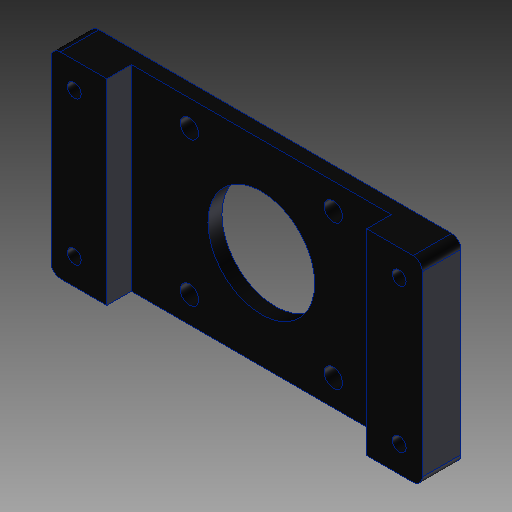
# Autodesk Inventor part: 3217a_Stepper Motor Plate_V1
Saved by Autodesk Inventor 2020 (Build 240168000, 168)
## iProperties
Created: 2019-11-01
Part Number: 3217a_Stepper Motor Plate_V1
Material: Aluminum 6061
Document SubType Name: Modeling
Designer: RFLab
Density: 2.7 g/cm^3
Appearance: Aluminum - Flat
Mass: 37.4548 g
Surface Area: 83.1003 cm^2
Volume: 13.8722 cm^3
Author: RFLab
Autodesk Inventor part; units mm, degrees
ref_plane "YZ Plane" through (0, 0, 0) normal (1, 0, 0) x (0, 1, 0)
ref_plane "XZ Plane" through (0, 0, 0) normal (0, 1, 0) x (-1, 0, 0)
ref_plane "XY Plane" through (0, 0, 0) normal (0, 0, 1) x (1, 0, 0)
sketch "Sketch1" plane through (0, 0, 0) normal (0, 0, 1) x (1, 0, 0)
  line L0 (-40, -21.15) -> (40, -21.15)
  line L1 (40, -21.15) -> (40, 21.15)
  line L2 (40, 21.15) -> (-40, 21.15)
  line L3 (-40, 21.15) -> (-40, -21.15)
  line L4 (-15.5, -15.5) -> (15.5, -15.5) construction
  line L5 (15.5, -15.5) -> (15.5, 15.5) construction
  line L6 (15.5, 15.5) -> (-15.5, 15.5) construction
  line L7 (-15.5, 15.5) -> (-15.5, -15.5) construction
  line L8 (-15.5, -15.5) -> (15.5, 15.5) construction
  line L9 (15.5, -15.5) -> (-15.5, 15.5) construction
  circle A0 centre (-15.5, 15.5) radius 2
  circle A1 centre (15.5, 15.5) radius 2
  circle A2 centre (15.5, -15.5) radius 2
  circle A3 centre (-15.5, -15.5) radius 2
  circle A4 centre (-35, 15.5) radius 1.5
  circle A5 centre (-35, -15.5) radius 1.5
  circle A6 centre (35, -15.5) radius 1.5
  circle A7 centre (35, 15.5) radius 1.5
  circle A8 centre (0, 0) radius 11.5
  point P0 (-40, 0)
  point P1 (0, 21.15)
  dimension "d0" = 80
  dimension "d1" = 42.3
  dimension "d2" = 31
  dimension "d3" = 31
  dimension "d4" = 4
  dimension "d5" = 4
  dimension "d6" = 4
  dimension "d7" = 4
  dimension "d8" = 3
  dimension "d9" = 3
  dimension "d10" = 3
  dimension "d11" = 3
  dimension "d12" = 5
  dimension "d13" = 5
  dimension "d17" = 23
  constraints: 20 end point, 9 centre point, 5 coincident, 5 horizontal alignment, 4 midpoint, 4 parallel, 3 vertical alignment, 2 horizontal, 2 perpendicular
  measures "d0" distance of L1.end L2.end
  measures "d1" distance of L2.end L0.start
  measures "d2" distance of L6.end L5.end
  measures "d3" distance of L4.end L5.end
  measures "d4" diameter of A0
  measures "d5" diameter of A1
  measures "d6" diameter of A2
  measures "d7" diameter of A3
  measures "d8" diameter of A4
  measures "d9" diameter of A5
  measures "d10" diameter of A6
  measures "d11" diameter of A7
  measures "d12" distance from line of L3 A4.centre
  measures "d13" distance from line of L1 A7.centre
  measures "d17" diameter of A8
extrude "Extrusion1" add sketch "Sketch1" along normal mid plane 3
fillet "Fillet1" radius 2 4 edges at (-40, -21.15, 0) (-40, 21.15, 0) (40, -21.15, 0) (40, 21.15, 0)
sketch "Sketch2" plane through (0, 0, 1.5) normal (0, 0, 1) x (1, 0, 0)
  arc A0 (40, 19.15) -> (38, 21.15) centre (38, 19.15) ccw projected
  line L0 (38, 21.15) -> (-38, 21.15) projected
  arc A1 (-38, 21.15) -> (-40, 19.15) centre (-38, 19.15) ccw projected
  line L1 (-40, 19.15) -> (-40, -19.15) projected
  arc A2 (-40, -19.15) -> (-38, -21.15) centre (-38, -19.15) ccw projected
  line L2 (-38, -21.15) -> (38, -21.15) projected
  arc A3 (38, -21.15) -> (40, -19.15) centre (38, -19.15) ccw projected
  line L3 (40, -19.15) -> (40, 19.15) projected
  circle A4 centre (0, 0) radius 11.5 projected
  circle A5 centre (-15.5, 15.5) radius 2 projected
  circle A6 centre (15.5, 15.5) radius 2 projected
  circle A7 centre (15.5, -15.5) radius 2 projected
  circle A8 centre (-15.5, -15.5) radius 2 projected
  circle A9 centre (-35, 15.5) radius 1.5 projected
  circle A10 centre (-35, -15.5) radius 1.5 projected
  circle A11 centre (35, -15.5) radius 1.5 projected
  circle A12 centre (35, 15.5) radius 1.5 projected
  line L4 (-38, -21.15) -> (38, -21.15) projected
  line L5 (-28, -21.15) -> (28, -21.15)
  line L6 (28, -21.15) -> (28, 21.15)
  line L7 (28, 21.15) -> (-28, 21.15)
  line L8 (-28, 21.15) -> (-28, -21.15)
  point P0 (-28, 21.15)
  dimension "d18" = 12
  dimension "d19" = 12
  constraints: 8 end point, 2 parallel, 2 point on line, 1 horizontal, 1 perpendicular
  measures "d18" distance between parallel lines of L1 L8
  measures "d19" distance between parallel lines of L3 L6
extrude "Extrusion2" add sketch "Sketch2" along normal blind 5.3 contours L3 A3 L2 L6 L0 A0 | L8 L2 A2 L1 A1 L0
body "Solid1"
